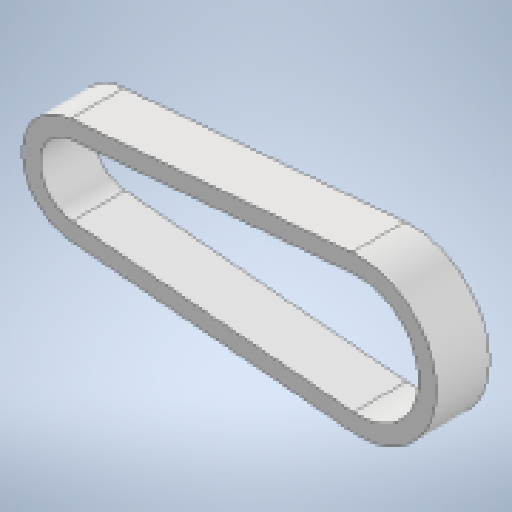
# Autodesk Inventor part: adapter
Saved by Autodesk Inventor 2025.2 (Build 292293000, 293)
## iProperties
Created: 2026-05-11
Part Number: adapter
Material: Ogólny
Document SubType Name: Modeling
Designer: muszy
Density: 1 g/cm^3
Appearance: Domyślna
Author: muszy
Autodesk Inventor part; units mm, degrees
ref_plane "YZ Plane" through (0, 0, 0) normal (1, 0, 0) x (0, 1, 0)
ref_plane "XZ Plane" through (0, 0, 0) normal (0, 1, 0) x (-1, 0, 0)
ref_plane "XY Plane" through (0, 0, 0) normal (0, 0, 1) x (1, 0, 0)
sketch "Szkic1" plane through (0, 0, 0) normal (0, 0, 1) x (1, 0, 0)
  line L0 (6.7664, -3.387) -> (-9.1111, -1.9923) projected
  arc A0 (6.7664, 3.387) -> (6.7664, -3.387) centre (7.0639, 0) ccw construction
  line L1 (6.7664, 3.387) -> (-9.1111, 1.9923) projected
  arc A1 (-9.1111, 1.9923) -> (-9.1111, -1.9923) centre (-8.9361, 0) ccw projected
  circle A2 centre (-5.2361, 0) radius 0.5 projected
  circle A3 centre (-7.1361, 0) radius 0.5 projected
  circle A4 centre (-9.0361, 0) radius 0.5 projected
  circle A5 centre (2.3639, 0) radius 0.5 projected
  circle A6 centre (0.4639, 0) radius 0.5 projected
  circle A7 centre (-1.4361, 0) radius 0.5 projected
  circle A8 centre (-3.3361, 0) radius 0.5 projected
  circle A9 centre (7.0639, 0) radius 3.4 construction
  arc A10 (6.6789, -4.3831) -> (6.6789, 4.3831) centre (7.0639, 0) ccw
  line L2 (6.7664, 3.387) -> (-9.1111, 1.9923) projected
  line L3 (6.7664, -3.387) -> (-9.1111, -1.9923) projected
  arc A11 (-9.1111, 1.9923) -> (-9.1111, -1.9923) centre (-8.9361, 0) ccw projected
  arc A12 (-9.1986, 2.9885) -> (-9.1986, -2.9885) centre (-8.9361, 0) ccw
  line L4 (-9.1986, -2.9885) -> (6.6789, -4.3831)
  line L5 (-9.1986, 2.9885) -> (6.6789, 4.3831)
  circle A13 centre (7.0639, 0) radius 3.4 projected
  line L6 (6.7664, 3.387) -> (-9.1111, 1.9923) projected
  line L7 (6.7664, -3.387) -> (-9.1111, -1.9923) projected
  arc A14 (-9.1111, 1.9923) -> (-9.1111, -1.9923) centre (-8.9361, 0) ccw projected
  dimension "d1" = 1
  constraints: 4 end point, 4 point on circle, 2 centre point, 3 other
  measures "d1" radial gap between concentric circles of A1 A12
extrude "Wyciągnięcie proste1" add sketch "Szkic1" along normal blind 3 contours L0 A1 L1 A13 | A13 | A2 | A3 | A4 | A5 | A6 | A7 | A8 | L4 A12 L5 A10
sketch "Szkic2" plane through (0, 0, 3) normal (0, 0, 1) x (1, 0, 0)
  circle A0 centre (7.0639, 0) radius 3.4 projected
  arc A1 (-9.1111, 1.9923) -> (-9.1111, -1.9923) centre (-8.9361, 0) ccw projected
  line L0 (6.7664, -3.387) -> (-9.1111, -1.9923) projected
  line L1 (6.7664, 3.387) -> (-9.1111, 1.9923) projected
  point P0 (0, 0)
extrude "Wyciągnięcie proste2" cut sketch "Szkic2" against normal blind 3
